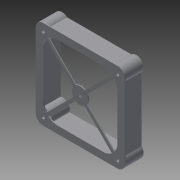
# Autodesk Inventor part: motorSupportSpacer
Saved by Autodesk Inventor 2014 SP2 (Build 180246200, 246)
## iProperties
Created: 2020-04-08
Part Number: motorSupportSpacer
Material: Generic
Document SubType Name: Sheet Metal
Designer: GauchoHP
Density: 1 g/cm^3
Sheet Metal Rule: Default_mm
Appearance: Default
Author: GauchoHP
Autodesk Inventor part; units mm, degrees
ref_plane "YZ Plane" through (0, 0, 0) normal (1, 0, 0) x (0, 1, 0)
ref_plane "XZ Plane" through (0, 0, 0) normal (0, 1, 0) x (-1, 0, 0)
ref_plane "XY Plane" through (0, 0, 0) normal (0, 0, 1) x (1, 0, 0)
sketch "Sketch1" plane through (0, 0, 0) normal (0, 1, 0) x (-1, 0, 0)
  circle A0 centre (0, 0) radius 1.5
  line L0 (-36, 43) -> (36, 43)
  line L1 (43, 36) -> (43, -36)
  line L2 (36, -43) -> (-36, -43)
  line L3 (-43, -36) -> (-43, 36)
  circle A1 centre (36, 36) radius 1.75
  circle A2 centre (36, -36) radius 1.75
  circle A3 centre (-36, -36) radius 1.75
  arc A4 (-36, 43) -> (-43, 36) centre (-36, 36) ccw
  arc A5 (43, 36) -> (36, 43) centre (36, 36) ccw
  arc A6 (36, -43) -> (43, -36) centre (36, -36) ccw
  arc A7 (-43, -36) -> (-36, -43) centre (-36, -36) ccw
  circle A8 centre (-36, 36) radius 1.75
  line L4 (-36, 22) -> (-36, -22)
  line L5 (-22, -36) -> (22, -36)
  line L6 (36, -22) -> (36, 22)
  line L7 (22, 36) -> (-22, 36)
  line L8 (-36, 36) -> (36, -36)
  arc A9 (-22, 36) -> (-30.7818, 32.9032) centre (-22, 22) ccw
  arc A10 (-32.9032, 30.7818) -> (-36, 22) centre (-22, 22) ccw
  arc A11 (22, -36) -> (30.7818, -32.9032) centre (22, -22) ccw
  arc A12 (32.9032, -30.7818) -> (36, -22) centre (22, -22) ccw
  line L9 (-36, -36) -> (36, 36)
  arc A13 (36, 22) -> (32.9032, 30.7818) centre (22, 22) ccw
  arc A14 (30.7818, 32.9032) -> (22, 36) centre (22, 22) ccw
  arc A15 (-36, -22) -> (-32.9032, -30.7818) centre (-22, -22) ccw
  arc A16 (-30.7818, -32.9032) -> (-22, -36) centre (-22, -22) ccw
  line L10 (-32.9032, -30.7818) -> (-6.6172, -4.4959)
  line L11 (-32.9032, 30.7818) -> (-6.6172, 4.4959)
  arc A17 (-6.6172, 4.4959) -> (-6.6172, -4.4959) centre (0, 0) ccw
  line L12 (-30.7818, 32.9032) -> (-4.4959, 6.6172)
  line L13 (-1.4489, -0.3882) -> (0.3882, 1.4489)
  line L14 (4.4959, 6.6172) -> (30.7818, 32.9032)
  arc A18 (4.4959, 6.6172) -> (-4.4959, 6.6172) centre (0, 0) ccw
  line L15 (-30.7818, -32.9032) -> (-4.4959, -6.6172)
  line L16 (-1.4489, 0.3882) -> (0.3882, -1.4489)
  line L17 (4.4959, -6.6172) -> (30.7818, -32.9032)
  arc A19 (-4.4959, -6.6172) -> (4.4959, -6.6172) centre (0, 0) ccw
  arc A20 (6.6172, -4.4959) -> (6.6172, 4.4959) centre (0, 0) ccw
  line L18 (-0.3882, 1.4489) -> (1.4489, -0.3882)
  line L19 (6.6172, -4.4959) -> (32.9032, -30.7818)
  line L20 (-0.3882, -1.4489) -> (1.4489, 0.3882)
  line L21 (6.6172, 4.4959) -> (32.9032, 30.7818)
  point P0 (-43, 43)
  point P1 (43, -43)
  point P2 (43, 43)
  point P3 (-43, -43)
  dimension "d0" = 3
  dimension "d1" = 86
  dimension "d2" = 86
  dimension "d3" = 43
  dimension "d4" = 43
  dimension "d9" = 3.5
  dimension "d11" = 3.5
  dimension "d12" = 3.5
  dimension "d20" = 7
  dimension "d25" = 3.5
  dimension "d26" = 7
  dimension "d27" = 7
  dimension "d29" = 7
  dimension "d30" = 7
  dimension "d31" = 7
  dimension "d32" = 7
  dimension "d33" = 7
  dimension "d34" = 7
  dimension "d35" = 72
  dimension "d50" = 7
  constraints: 44 end point, 32 point on circle, 20 centre point, 16 parallel, 16 tangent, 8 point on line, 3 coincident, 3 equal radius, 2 perpendicular, 1 horizontal, 13 other
  measures "d1" distance of point (43, -43) point (-43, -43)
  measures "d2" distance of point (43, 43) point (43, -43)
  measures "d3" distance from line of point (0, 0) L3
  measures "d4" distance from line of point (0, 0) L0
  measures "d9" diameter of A1
  measures "d11" diameter of A2
  measures "d12" diameter of A3
  measures "d20" radius of A4
  measures "d25" diameter of A8
  measures "d26" distance from line of L1 L9.end
  measures "d27" distance from line of L0 L9.end
  measures "d29" distance from line of A4.centre L3
  measures "d30" distance from line of L0 A4.centre
  measures "d31" distance from line of L9.start L3
  measures "d32" distance from line of A3.centre L2
  measures "d33" distance from line of L2 L8.end
  measures "d34" distance from line of L1 L8.end
  measures "d35" distance of A4.centre A3.centre
  measures "d50" distance between parallel lines of L4 L3
extrude "Extrusion1" add sketch "Sketch1" along normal blind 1
sketch "Sketch3" plane through (0, 1, 0) normal (0, 1, 0) x (1, 0, 0)
  circle A0 centre (36, -36) radius 1.75 projected
  circle A1 centre (36, 36) radius 1.75 projected
  circle A2 centre (-36, 36) radius 1.75 projected
  circle A3 centre (-36, -36) radius 1.75 projected
  line L0 (-36, -43) -> (36, -43) projected
  arc A4 (36, -43) -> (43, -36) centre (36, -36) ccw projected
  line L1 (43, -36) -> (43, 36) projected
  arc A5 (43, 36) -> (36, 43) centre (36, 36) ccw projected
  line L2 (36, 43) -> (-36, 43) projected
  arc A6 (-36, 43) -> (-43, 36) centre (-36, 36) ccw projected
  line L3 (-43, 36) -> (-43, -36) projected
  arc A7 (-43, -36) -> (-36, -43) centre (-36, -36) ccw projected
  circle A8 centre (-36, 36) radius 7
  circle A9 centre (36, 36) radius 7
  circle A10 centre (36, -36) radius 7
  circle A11 centre (-36, -36) radius 7
  line L4 (-38, 29.2918) -> (-38, -29.2918)
  line L5 (-29.2918, 38) -> (29.2918, 38)
  line L6 (38, 29.2918) -> (38, -29.2918)
  line L7 (29.2918, -38) -> (-29.2918, -38)
  line L8 (-41, 31.101) -> (-41, -31.101)
  line L9 (41, 31.101) -> (41, -31.101)
  line L10 (-31.101, 41) -> (31.101, 41)
  line L11 (-31.101, -41) -> (31.101, -41)
  dimension "d36" = 5
  dimension "d37" = 5
  dimension "d38" = 5
  dimension "d39" = 5
  dimension "d40" = 76
  dimension "d41" = 76
  dimension "d42" = 3
  dimension "d43" = 3
  dimension "d44" = 3
  dimension "d45" = 3
  constraints: 19 point on circle, 16 end point, 5 perpendicular, 4 centre point, 4 coincident, 3 parallel, 1 concentric
  measures "d36" distance between parallel lines of L4 L3
  measures "d37" distance between parallel lines of L1 L6
  measures "d38" distance between parallel lines of L0 L7
  measures "d39" distance between parallel lines of L2 L5
  measures "d40" distance between parallel lines of L6 L4
  measures "d41" distance between parallel lines of L7 L5
  measures "d42" distance between parallel lines of L8 L4
  measures "d43" distance between parallel lines of L9 L6
  measures "d44" distance between parallel lines of L10 L5
  measures "d45" distance between parallel lines of L11 L7
extrude "Extrusion2" add sketch "Sketch3" along normal blind 18 contours A7 A11 | A10 A4 | A11 L7 A10 L11 | A6 A8 | L8 A8 L4 A11 | A9 A5 | A10 L6 A9 L9 | L10 A9 L5 A8
fillet "Fillet2" radius 1 8 edges at (-40.9497, 19, -40.9497) (40.9497, 19, -40.9497) (40.9497, 19, 40.9497) (-40.9497, 19, 40.9497) (-41, 19, 0) (0, 19, 41) (41, 19, 0) (0, 19, -41)
chamfer "Chamfer2" distance 0.93 angle 45 2 edges at (33.056, 1, -29.6492) (29.6492, 1, -33.056)
chamfer "Chamfer3" distance 0.93 angle 45 2 edges at (33.056, 1, 29.6492) (29.6492, 1, 33.056)
chamfer "Chamfer4" distance 0.93 angle 45 2 edges at (-29.6492, 1, -33.056) (-33.056, 1, -29.6492)
chamfer "Chamfer5" distance 0.93 angle 45 2 edges at (-33.056, 1, 29.6492) (-29.6492, 1, 33.056)
chamfer "Chamfer6" distance 6 distance2 0.5 1 edges at (1.5, 1, 0)
equation "\"BendRadius\" = Thickness"
equation "\"BendReliefWidth\" = Thickness"
equation "\"BendReliefDepth\" = 0.5 * Thickness"
equation "\"CornerReliefSize\" = 4 * Thickness"
equation "\"MinimumRemnant\" = 2 * Thickness"
equation "\"TransitionRadius\" = BendRadius"
equation "\"JacobiRadiusSize\" = BendRadius"
equation "\"GapSize\" = Thickness"
equation "\"Thickness\" = 0.5"
body "Solid1"
